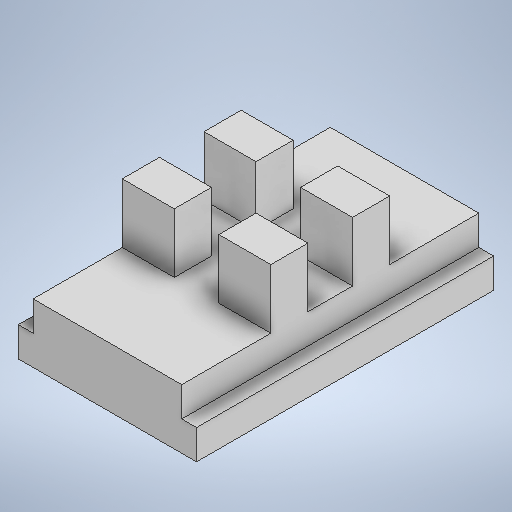
# Autodesk Inventor part: 18
Saved by Autodesk Inventor 2025.1 (Build 291241000, 241)
## iProperties
Created: 2024-09-13
Part Number: 18
Material: Generisch
Document SubType Name: Modeling
Designer: ffogue
Density: 1 g/cm^3
Appearance: Vorgabe
Author: ffogue
Autodesk Inventor part; units mm, degrees
ref_plane "YZ Plane" through (0, 0, 0) normal (1, 0, 0) x (0, 1, 0)
ref_plane "XZ Plane" through (0, 0, 0) normal (0, 1, 0) x (-1, 0, 0)
ref_plane "XY Plane" through (0, 0, 0) normal (0, 0, 1) x (1, 0, 0)
sketch "Sketch1" plane through (0, 0, 0) normal (0, 0, 1) x (1, 0, 0)
  line L0 (-6, -10) -> (6, -10)
  line L1 (6, -10) -> (6, 10)
  line L2 (6, 10) -> (-6, 10)
  line L3 (-6, 10) -> (-6, -10)
  line L4 (-6, -10) -> (6, 10) construction
  line L5 (6, -10) -> (-6, 10) construction
  point P0 (0, 0)
  dimension "d0" = 12
  dimension "d1" = 20
  constraints: 12 end point, 2 midpoint, 2 parallel, 1 horizontal, 1 perpendicular
  measures "d0" distance of L1.end L2.end
  measures "d1" distance of L2.end L0.start
extrude "Extrusion1" add sketch "Sketch1" along normal blind 2
sketch "Sketch2" plane through (0, 0, 2) normal (0, 0, 1) x (1, 0, 0)
  line L0 (-5, -10) -> (5, -10)
  line L1 (5, -10) -> (5, 10)
  line L2 (5, 10) -> (-5, 10)
  line L3 (-5, 10) -> (-5, -10)
  line L4 (-5, -10) -> (5, 10) construction
  line L5 (5, -10) -> (-5, 10) construction
  point P0 (0, 0)
  point P1 (-6, 10)
  dimension "d4" = 10
  constraints: 12 end point, 2 midpoint, 2 parallel, 1 horizontal, 1 horizontal alignment, 1 perpendicular
  measures "d4" distance of L1.end L2.end
extrude "Extrusion2" add sketch "Sketch2" along normal blind 2
sketch "Sketch3" plane through (0, 0, 4) normal (0, 0, 1) x (1, 0, 0)
  line L0 (-5, 10) -> (-5, -10) projected
  line L1 (-5, 4) -> (-1.5, 4)
  line L2 (-1.5, 4) -> (-1.5, 1.5)
  line L3 (-1.5, 1.5) -> (-5, 1.5)
  line L4 (-5, -1.5) -> (-1.5, -1.5)
  line L5 (-1.5, -1.5) -> (-1.5, -4)
  line L6 (-1.5, -4) -> (-5, -4)
  line L7 (5, 10) -> (-5, 10) projected
  line L8 (-5, -10) -> (5, -10) projected
  point P0 (0, 0)
  dimension "d7" = 6
  dimension "d8" = 2.5
  dimension "d9" = 6
  dimension "d10" = 2.5
  dimension "d11" = 1.5
  constraints: 12 end point, 5 point on line, 3 parallel, 2 perpendicular, 1 horizontal
  measures "d7" distance between parallel lines of L7 L1
  measures "d8" distance of L1.end L2.end
  measures "d9" distance between parallel lines of L8 L6
  measures "d10" distance of L4.end L5.end
  measures "d11" distance from line of point (0, 0) L2
extrude "Extrusion3" add sketch "Sketch3" along normal blind 4
mirror "Mirror1" about plane through (0, 0, 0) normal (1, 0, 0) of "Extrusion3"
sketch "Sketch4" plane through (0, 0, 0) normal (0, 0, -1) x (-1, 0, 0)
  line L0 (-3.5, -6.25) -> (3.5, -6.25)
  line L1 (3.5, -6.25) -> (3.5, 6.25)
  line L2 (3.5, 6.25) -> (-3.5, 6.25)
  line L3 (-3.5, 6.25) -> (-3.5, -6.25)
  line L4 (-3.5, -6.25) -> (3.5, 6.25) construction
  line L5 (3.5, -6.25) -> (-3.5, 6.25) construction
  line L6 (-6, 10) -> (6, 10) projected
  point P0 (0, 0)
  dimension "d14" = 12.5
  dimension "d15" = 3.75
  dimension "d16" = 7
  constraints: 12 end point, 2 midpoint, 2 parallel, 1 horizontal, 1 perpendicular
  measures "d14" distance of L2.end L0.start
  measures "d15" distance between parallel lines of L6 L2
  measures "d16" distance of L1.end L2.end
extrude "Extrusion4" cut sketch "Sketch4" against normal blind 3
equation "\"d9\" = d7"
equation "\"d10\" = d8"
body "Solid1"
